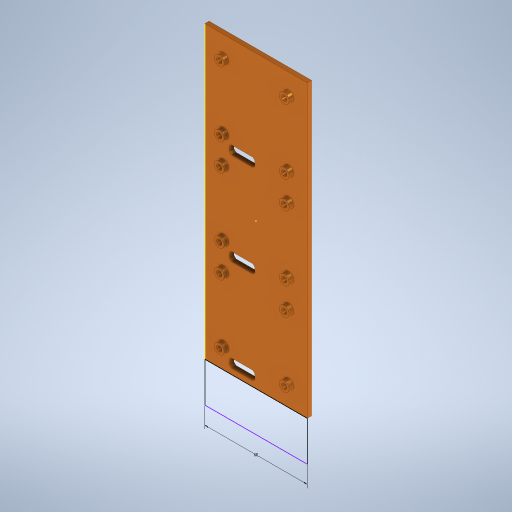
# Autodesk Inventor part: BasePotencia
Saved by Autodesk Inventor 2024.2 (Build 282272000, 272)
## iProperties
Created: 2024-08-03
Part Number: BasePotencia
Material: Gold
Document SubType Name: Modeling
Designer: Admin
Density: 19.3 g/cm^3
Appearance: Metal 1600F Hot
Author: Admin
Autodesk Inventor part; units mm, degrees
ref_plane "YZ Plane" through (0, 0, 0) normal (1, 0, 0) x (0, 1, 0)
ref_plane "XZ Plane" through (0, 0, 0) normal (0, 1, 0) x (-1, 0, 0)
ref_plane "XY Plane" through (0, 0, 0) normal (0, 0, 1) x (1, 0, 0)
sketch "Sketch1" plane through (0, 0, 0) normal (0, 0, 1) x (1, 0, 0)
  line L0 (-30, -85) -> (30, -85)
  line L1 (30, -85) -> (30, 85)
  line L2 (30, 85) -> (-30, 85)
  line L3 (-30, 85) -> (-30, -85)
  line L4 (-30, -85) -> (30, 85) construction
  line L5 (30, -85) -> (-30, 85) construction
  line L6 (-19, 19) -> (19, 19)
  line L7 (19, 19) -> (19, -19)
  line L8 (19, -19) -> (-19, -19)
  line L9 (-19, -19) -> (-19, 19)
  line L10 (-19, 19) -> (19, -19) construction
  line L11 (19, 19) -> (-19, -19) construction
  circle A0 centre (19, 19) radius 1.5875
  circle A1 centre (19, 19) radius 3
  circle A2 centre (-19, 19) radius 3
  circle A3 centre (-19, 19) radius 1.5875
  circle A4 centre (-19, -19) radius 3
  circle A5 centre (-19, -19) radius 1.5875
  circle A6 centre (19, -19) radius 3
  circle A7 centre (19, -19) radius 1.5875
  circle A8 centre (19, -35) radius 3
  circle A9 centre (19, -35) radius 1.5875
  circle A10 centre (-19, -35) radius 1.5875
  circle A11 centre (-19, -35) radius 3
  circle A12 centre (-19, -73) radius 3
  circle A13 centre (-19, -73) radius 1.5875
  circle A14 centre (19, -73) radius 3
  circle A15 centre (19, -73) radius 1.5875
  circle A16 centre (19, 73) radius 3
  circle A17 centre (19, 73) radius 1.5875
  circle A18 centre (-19, 73) radius 1.5875
  circle A19 centre (-19, 73) radius 3
  circle A20 centre (-19, 35) radius 3
  circle A21 centre (-19, 35) radius 1.5875
  circle A22 centre (19, 35) radius 3
  circle A23 centre (19, 35) radius 1.5875
  circle A24 centre (19, 19) radius 3
  circle A25 centre (19, 19) radius 1.5875
  circle A26 centre (-19, 19) radius 1.5875
  circle A27 centre (-19, 19) radius 3
  circle A28 centre (-19, -19) radius 3
  circle A29 centre (-19, -19) radius 1.5875
  circle A30 centre (19, -19) radius 3
  circle A31 centre (19, -19) radius 1.5875
  point P0 (0, 0)
  dimension "d0" = 170
  dimension "d1" = 60
  dimension "d2" = 38
  dimension "d3" = 38
  dimension "d6" = 6
  dimension "d7" = 3.175
  dimension "d10" = 360
  dimension "d14" = 54
  dimension "d17" = 54
  constraints: 32 centre point, 24 end point, 17 coincident, 4 midpoint, 4 parallel, 2 horizontal, 2 perpendicular, 2 vertical, 65 other
  measures "d0" distance of L2.end L0.start
  measures "d1" distance of L1.end L2.end
  measures "d2" distance of L7.end L8.end
  measures "d3" distance of L6.end L7.end
  measures "d6" diameter of A1
  measures "d7" diameter of A0
  measures "d14" distance of A1.centre A8.centre
  measures "d17" distance of A1.centre A16.centre
extrude "Extrusion1" add sketch "Sketch1" along normal blind 2.5 contours L3 L2 L1 L0 | L6 A1 L7 A6 L8 A4 L9 A2
extrude "Extrusion2" add sketch "Sketch1" along normal blind 5 contours A3 L9 A2 L6 | L6 A2 L9 A3 | A1 L7 A0 L6 | L6 A0 L7 A1 | A4 L8 A5 L9 | L9 A5 L8 A4 | A6 L8 A7 L7 | L7 A7 L8 A6 | A8 | A11 | A12 | A14 | A16 | A19 | A20 | A22
sketch "Sketch2" plane through (0, 0, 2.5) normal (0, 0, 1) x (1, 0, 0)
  line L0 (-15.4, 31.4) -> (-0.6, 31.4)
  line L1 (-0.6, 31.4) -> (-0.6, 26.4)
  line L2 (-0.6, 26.4) -> (-15.4, 26.4)
  line L3 (-15.4, 26.4) -> (-15.4, 31.4)
  circle A0 centre (-19, 35) radius 1.5875 projected
  line L4 (-19, 35) -> (-15.4, 31.4)
  line L5 (-19, 35) -> (-14, 35)
  line L6 (-30, 85) -> (-30, -85) projected
  line L7 (-30, 0) -> (-30, 23)
  line L8 (-15.4, -22.6) -> (-0.6, -22.6)
  line L9 (-0.6, -22.6) -> (-0.6, -27.6)
  line L10 (-0.6, -27.6) -> (-15.4, -27.6)
  line L11 (-15.4, -27.6) -> (-15.4, -22.6)
  line L12 (-15.4, -76.6) -> (-0.6, -76.6)
  line L13 (-0.6, -76.6) -> (-0.6, -81.6)
  line L14 (-0.6, -81.6) -> (-15.4, -81.6)
  line L15 (-15.4, -81.6) -> (-15.4, -76.6)
  line L16 (-14.2, 31.4) -> (-15.4, 30.2)
  line L17 (-8, 26.4) -> (-8, 31.4)
  line L18 (-0.6, 28.9) -> (-8, 28.9)
  line L19 (-1.8, 31.4) -> (-0.6, 30.2)
  line L20 (-14.2, 26.4) -> (-15.4, 27.6)
  line L21 (-1.8, 26.4) -> (-0.6, 27.6)
  line L22 (-14.2, -22.6) -> (-15.4, -23.8)
  line L23 (-1.8, -22.6) -> (-0.6, -23.8)
  line L24 (-1.8, -27.6) -> (-0.6, -26.4)
  line L25 (-14.2, -27.6) -> (-15.4, -26.4)
  line L26 (-14.2, -76.6) -> (-15.4, -77.8)
  line L27 (-1.8, -76.6) -> (-0.6, -77.8)
  line L28 (-1.8, -81.6) -> (-0.6, -80.4)
  line L29 (-14.2, -81.6) -> (-15.4, -80.4)
  point P0 (0, 0)
  point P1 (-15.4, -80.4)
  point P2 (-0.6, -80.4)
  point P3 (-0.6, -77.8)
  point P4 (-15.4, -77.8)
  point P5 (-15.4, -26.4)
  point P6 (-0.6, -26.4)
  point P7 (-0.6, -23.8)
  point P8 (-15.4, -23.8)
  point P9 (-15.4, 27.6)
  point P10 (-0.6, 27.6)
  point P11 (-0.6, 30.2)
  dimension "d24" = 5
  dimension "d25" = 45
  dimension "d26" = 14.8
  dimension "d27" = 5
  dimension "d31" = 54
  dimension "d38" = 3.6
  dimension "d39" = 135
  dimension "d40" = 1.2
  dimension "d43" = 54
  constraints: 58 end point, 6 symmetric about line, 5 midpoint, 3 point on line, 2 horizontal, 2 parallel, 2 vertical, 1 perpendicular, 40 other
  measures "d24" distance of L4.start L5.end
  measures "d25" angle of L4 L5
  measures "d26" distance of L0.start L0.end
  measures "d27" distance of L2.end L0.start
  measures "d31" distance of L0.start L8.start
  measures "d38" distance from line of L4.start L3
  measures "d39" angle of L0 L16
  measures "d40" horizontal distance of L16.start L16.end
  measures "d43" distance of L16.start L22.start
extrude "Extrusion3" cut sketch "Sketch2" against normal blind 5 contours L0 L17 L2 L20 L3 L16 | L0 L19 L1 L18 L17 | L18 L1 L21 L2 L17 | L8 L23 L9 L24 L10 L25 L11 L22 | L12 L27 L13 L28 L14 L29 L15 L26
sketch "Sketch4" plane through (0, 0, 2.5) normal (0, 0, 1) x (1, 0, 0)
  line L0 (-30, 85) -> (-30, -85) projected
  line L1 (-30, -85) -> (30, -85)
  line L2 (30, -85) -> (30, -108.2556)
  line L3 (30, -108.2556) -> (-30, -108.2556)
  line L4 (-30, -108.2556) -> (-30, -85)
  point P0 (0, 0)
  dimension "d54" = 60
  constraints: 8 end point, 2 parallel, 1 horizontal, 1 perpendicular
  measures "d54" distance of L2.end L3.end
body "Solid1"
